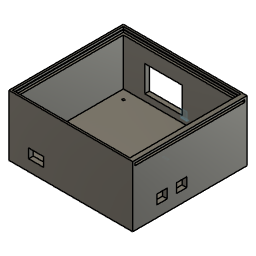
Shades+PCB+Holder+#1 (Autodesk Fusion 360 design; units mm, degrees)
Autodesk Fusion 360 part; units mm, degrees
sketch "Sketch1" plane through (0, 0, 0) normal (0, 1, 0) x (1, 0, 0)
  line L0 (0, 0) -> (132.5, 0)
  line L1 (132.5, 0) -> (132.5, 122.5)
  line L2 (132.5, 122.5) -> (0, 122.5)
  line L3 (0, 122.5) -> (0, 0)
  line L4 (127.5, 117.5) -> (5, 117.5)
  line L5 (5, 117.5) -> (5, 5)
  line L6 (5, 5) -> (127.5, 5)
  line L7 (127.5, 5) -> (127.5, 117.5)
  constraint coincident L0.start L3.end
  constraint horizontal L0
  constraint perpendicular L0 L1
  constraint perpendicular L1 L2
  constraint perpendicular L0 L3
  constraint horizontal L4
  constraint vertical L5
  constraint horizontal L6
  constraint vertical L7
extrude "Extrude1" add sketch "Sketch1" along normal blind 5 contours L0 L1 L2 L3 | L4 L5 L6 L7
sketch "Sketch2" plane through (0, 5, 0) normal (0, 1, 0) x (-1, 0, 0)
  line L0 (0, -122.5) -> (0, 0)
  line L1 (0, 0) -> (-132.5, 0)
  line L2 (-132.5, 0) -> (-132.5, -122.5)
  line L3 (-132.5, -122.5) -> (0, -122.5)
  line L4 (0, -122.5) -> (-5, -122.5)
  line L5 (-132.5, 0) -> (-127.5, 0)
  line L6 (-5, -117.5) -> (-127.5, -117.5)
  line L7 (-127.5, -117.5) -> (-127.5, -5)
  line L8 (-127.5, -5) -> (-5, -5)
  line L9 (-5, -5) -> (-5, -117.5)
  dimension "d19" = 5
  dimension "d20" = 5
  constraint coincident L0.start L3.end
  constraint coincident L3 L4.end
  constraint perpendicular L0 L4
  constraint coincident L1.end L2.start
  constraint perpendicular L2 L5
  constraint horizontal L6
  constraint vertical L7
  constraint horizontal L8
  constraint vertical L9
  measures "d19" distance of L4.end L6.start
  measures "d20" distance of L1.end L5.end
extrude "Extrude2" add sketch "Sketch2" along normal blind 25
sketch "Sketch3" plane through (132.5, 0, 0) normal (1, 0, 0) x (0, 0, -1)
  line L0 (0, 0) -> (122.5, 0)
  line L1 (122.5, 0) -> (122.5, 30)
  line L2 (122.5, 30) -> (0, 30)
  line L3 (0, 30) -> (0, 0)
  circle A0 centre (20, 15) radius 2.5
  circle A1 centre (35, 15) radius 2.5
  line L4 (20, 15) -> (20, 17.5)
  line L5 (20, 17.5) -> (16, 17.5)
  line L6 (20, 15) -> (20, 12.5)
  line L7 (20, 12.5) -> (24, 12.5)
  line L8 (16, 17.5) -> (24, 17.5)
  line L9 (24, 17.5) -> (24, 12.5)
  line L10 (24, 12.5) -> (16, 12.5)
  line L11 (16, 12.5) -> (16, 17.5)
  line L12 (35, 15) -> (35, 17.5)
  line L13 (35, 17.5) -> (31, 17.5)
  line L14 (35, 12.5) -> (39, 12.5)
  line L15 (31, 17.5) -> (39, 17.5)
  line L16 (39, 17.5) -> (39, 12.5)
  line L17 (39, 12.5) -> (31, 12.5)
  line L18 (31, 12.5) -> (31, 17.5)
  line L19 (0, 30) -> (0, 27.5)
  line L20 (0, 27.5) -> (2.5, 27.5)
  line L21 (2.5, 27.5) -> (2.5, 25)
  line L22 (122.5, 30) -> (122.5, 27.5)
  line L23 (122.5, 27.5) -> (120, 27.5)
  line L24 (120, 27.5) -> (120, 25)
  line L25 (120, 25) -> (2.5, 25)
  line L26 (2.5, 27.5) -> (120, 27.5)
  dimension "d23" = 5
  dimension "d24" = 5
  dimension "d58" = 2.5
  dimension "d59" = 2.5
  dimension "d60" = 2.5
  dimension "d61" = 2.5
  constraint coincident A0.centre L4.start
  constraint coincident A0 L4.end
  constraint perpendicular L2 L4
  constraint tangent A0 L5
  constraint coincident A0 L6.end
  constraint perpendicular L5 L6
  constraint tangent A0 L7
  constraint horizontal L8
  constraint vertical L9
  constraint horizontal L10
  constraint vertical L11
  constraint coincident A1.centre L12.start
  constraint coincident A1 L12.end
  constraint perpendicular L2 L12
  constraint tangent A1 L13
  constraint coincident A1 L14.start
  constraint tangent A1 L14
  constraint perpendicular L12 L14
  constraint horizontal L15
  constraint vertical L16
  constraint horizontal L17
  constraint vertical L18
  constraint coincident L2.end L3.start
  constraint perpendicular L2 L19
  constraint perpendicular L19 L20
  constraint perpendicular L20 L21
  constraint coincident L1.end L2.start
  constraint perpendicular L2 L22
  constraint perpendicular L22 L23
  constraint perpendicular L23 L24
  constraint perpendicular L24 L25
  measures "d23" diameter of A0
  measures "d24" diameter of A1
  measures "d58" distance of L2.end L19.end
  measures "d59" distance of L19.end L20.end
  measures "d60" distance of L1.end L22.end
  measures "d61" distance of L22.end L23.end
extrude "Extrude3" cut sketch "Sketch3" against normal blind 10 contours A1
extrude "Extrude4" cut sketch "Sketch3" against normal blind 10 contours A0 L4 L6 | A0 L4 L6
sketch "Sketch4" plane through (0, 0, 0) normal (0, 0, 1) x (1, 0, 0)
  line L0 (0, 0) -> (132.5, 0)
  line L1 (132.5, 0) -> (132.5, 30)
  line L2 (132.5, 30) -> (0, 30)
  line L3 (0, 30) -> (0, 0)
  circle A0 centre (15, 15) radius 3.75
  line L4 (15, 15) -> (15, 18.75)
  line L5 (15, 18.75) -> (10, 18.75)
  line L6 (15, 15) -> (15, 11.25)
  line L7 (15, 11.25) -> (20, 11.25)
  line L8 (10, 18.75) -> (20, 18.75)
  line L9 (20, 18.75) -> (20, 11.25)
  line L10 (20, 11.25) -> (10, 11.25)
  line L11 (10, 11.25) -> (10, 18.75)
  dimension "d29" = 7.5
  constraint coincident A0.centre L4.start
  constraint coincident A0 L4.end
  constraint perpendicular L2 L4
  constraint tangent A0 L5
  constraint coincident A0 L6.end
  constraint perpendicular L5 L6
  constraint tangent A0 L7
  constraint horizontal L8
  constraint vertical L9
  constraint horizontal L10
  constraint vertical L11
  measures "d29" diameter of A0
extrude "Extrude5" cut sketch "Sketch4" against normal blind 10 contours A0 L4 L6 | A0 L4 L6
sketch "Sketch5" plane through (0, 5, 0) normal (0, 1, 0) x (-1, 0, 0)
  line L0 (-127.5, -5) -> (-127.5, -117.5)
  line L1 (-127.5, -117.5) -> (-5, -117.5)
  line L2 (-5, -117.5) -> (-5, -5)
  line L3 (-5, -5) -> (-127.5, -5)
  line L4 (-127.5, -117.5) -> (-86.9, -117.5)
  line L5 (-86.9, -117.5) -> (-86.9, -101.5)
  line L6 (-86.9, -101.5) -> (-86.9, -102.5)
  line L7 (-86.9, -102.5) -> (-84.4, -102.5)
  line L8 (-86.9, -101.5) -> (-86.9, -100.5)
  line L9 (-86.9, -100.5) -> (-89.4, -100.5)
  line L10 (-84.4, -102.5) -> (-89.4, -102.5)
  line L11 (-89.4, -102.5) -> (-89.4, -100.5)
  line L12 (-89.4, -100.5) -> (-84.4, -100.5)
  line L13 (-84.4, -100.5) -> (-84.4, -102.5)
  line L14 (-84.4, -102.5) -> (-83.4, -102.5)
  line L15 (-84.4, -100.5) -> (-83.4, -100.5)
  line L16 (-83.4, -102.5) -> (-83.4, -100.5)
  line L17 (-89.4, -102.5) -> (-90.4, -102.5)
  line L18 (-89.4, -100.5) -> (-90.4, -100.5)
  line L19 (-90.4, -102.5) -> (-90.4, -100.5)
  line L20 (-86.9, -101.5) -> (-86.9, -81)
  line L21 (-86.9, -81) -> (-86.9, -82)
  line L22 (-86.9, -81) -> (-86.9, -80)
  line L23 (-86.9, -82) -> (-83.9, -82)
  line L24 (-83.9, -82) -> (-83.9, -81)
  line L25 (-86.9, -82) -> (-89.9, -82)
  line L26 (-89.9, -82) -> (-89.9, -80)
  line L27 (-89.9, -80) -> (-83.9, -80)
  line L28 (-83.9, -80) -> (-83.9, -81)
  line L29 (-86.9, -81) -> (-86.9, -80)
  dimension "d32" = 40.6
  dimension "d36" = 16
  dimension "d37" = 1
  dimension "d38" = 2.5
  dimension "d39" = 1
  dimension "d40" = 2.5
  dimension "d41" = 1
  dimension "d42" = 1
  dimension "d43" = 1
  dimension "d44" = 1
  dimension "d45" = 20.5
  dimension "d46" = 1
  dimension "d47" = 3
  dimension "d48" = 3
  constraint coincident L0.end L1.start
  constraint perpendicular L0 L4
  constraint perpendicular L4 L5
  constraint vertical L6
  constraint perpendicular L5 L7
  constraint perpendicular L7 L8
  constraint perpendicular L8 L9
  constraint horizontal L10
  constraint vertical L11
  constraint horizontal L12
  constraint vertical L13
  constraint perpendicular L13 L14
  constraint perpendicular L13 L15
  constraint perpendicular L11 L17
  constraint perpendicular L11 L18
  constraint perpendicular L12 L20
  constraint parallel L20 L21
  constraint parallel L21 L22
  constraint perpendicular L20 L23
  constraint perpendicular L23 L24
  constraint perpendicular L20 L25
  constraint perpendicular L25 L26
  constraint perpendicular L26 L27
  constraint parallel L24 L28
  measures "d32" distance of L0.end L4.end
  measures "d36" distance of L4.end L5.end
  measures "d37" distance of L5.end L6.end
  measures "d38" distance of L6.end L7.end
  measures "d39" distance of L5.end L8.end
  measures "d40" distance of L8.end L9.end
  measures "d41" distance of L7.end L14.end
  measures "d42" distance of L12.end L15.end
  measures "d43" distance of L10.end L17.end
  measures "d44" distance of L9.end L18.end
  measures "d45" distance of L5.end L20.end
  measures "d46" distance of L20.end L21.end
  measures "d47" distance of L21.end L23.end
  measures "d48" distance of L21.end L25.end
extrude "Extrude6" add sketch "Sketch5" along normal blind 5 contours L0 L1 L2 L3 L4 | L5 L6 L8 L9 L10 L11 L12 L20 | L5 L6 L7 L8 L10 L12 L13 L20 | L13 L14 L15 L16 | L11 L17 L18 L19 | L20 L21 L22 L25 L26 L27 L29 | L20 L21 L22 L23 L24 L27 L28 L29
extrude "Extrude7" cut 1 faces at (86.6667, 10, -42.5) along direction (0, -1, 0) blind 5
move_face "OffsetFaces1" offset 5 1 faces at (44.1667, 0, -40.8333)
extrude "Extrude8" cut sketch "Sketch5" against normal blind 9 contours L5 L6 L8 L9 L10 L11 L12 L20 | L5 L6 L7 L8 L10 L12 L13 L20 | L13 L14 L15 L16 | L11 L17 L18 L19 | L20 L21 L22 L25 L26 L27 L29 | L20 L21 L22 L23 L24 L27 L28 L29
extrude "Extrude9" cut sketch "Sketch4" against normal blind 10 contours A0 L7 L8 L9 L10 | A0 L5 L8 L10 L11
extrude "Extrude10" cut sketch "Sketch3" against normal blind 15 contours A0 L7 L8 L9 L10 | A0 L5 L8 L10 L11 | A1 L14 L15 L16 L17 | A1 L13 L15 L17 L18
extrude "Extrude11" cut sketch "Sketch3" against normal blind 130 contours L21 L24 L25 L26
sketch "Sketch6" plane through (0, 5, 0) normal (0, 1, 0) x (-1, 0, 0)
  line L0 (-83.4, -100.5) -> (-83.4, -102.5)
  line L1 (-83.4, -102.5) -> (-90.4, -102.5)
  line L2 (-90.4, -102.5) -> (-90.4, -100.5)
  line L3 (-90.4, -100.5) -> (-83.4, -100.5)
  line L4 (-83.9, -80) -> (-83.9, -82)
  line L5 (-83.9, -82) -> (-89.9, -82)
  line L6 (-89.9, -82) -> (-89.9, -80)
  line L7 (-89.9, -80) -> (-83.9, -80)
  line L8 (-127.5, -117.5) -> (-5, -117.5)
  line L9 (-5, -117.5) -> (-5, -5)
  line L10 (-5, -5) -> (-127.5, -5)
  line L11 (-127.5, -5) -> (-127.5, -117.5)
  line L12 (-127.5, -117.5) -> (-117.5, -117.5)
  line L13 (-117.5, -117.5) -> (-117.5, -107.5)
  circle A0 centre (-117.5, -107.5) radius 1.25
  line L14 (-117.5, -107.5) -> (-117.5, -14.9)
  line L15 (-117.5, -14.9) -> (-15.1, -14.9)
  line L16 (-15.1, -14.9) -> (-15.1, -107.5)
  line L17 (-15.1, -107.5) -> (-117.5, -107.5)
  circle A1 centre (-117.5, -14.9) radius 1.25
  circle A2 centre (-15.1, -14.9) radius 1.25
  circle A3 centre (-15.1, -107.5) radius 1.25
  dimension "d64" = 10
  dimension "d65" = 10
  dimension "d66" = 2.5
  dimension "d67" = 92.6
  dimension "d68" = 102.4
  dimension "d69" = 92.6
  dimension "d70" = 2.5
  dimension "d71" = 2.5
  dimension "d72" = 2.5
  constraint coincident L8.start L11.end
  constraint perpendicular L11 L12
  constraint perpendicular L8 L13
  constraint coincident L13.end A0.centre
  constraint perpendicular L10 L14
  constraint perpendicular L14 L15
  constraint perpendicular L15 L16
  constraint coincident L14.end L15.start
  constraint coincident L15.end L16.start
  constraint coincident L16.end L17.start
  measures "d64" distance of L8.start L12.end
  measures "d65" distance of L12.end L13.end
  measures "d66" diameter of A0
  measures "d67" distance of L13.end L14.end
  measures "d68" distance of L14.end L15.end
  measures "d69" distance of L15.end L16.end
  measures "d70" diameter of A1
  measures "d71" diameter of A2
  measures "d72" diameter of A3
extrude "Extrude12" add sketch "Sketch6" along normal blind 90 contours L13 A0 L14 | L13 A0 L17 | A0 L14 L17 | L14 L15 A1 | L14 L15 A1 | L16 L17 A3 | L16 L17 A3 | L15 L16 A2 | L15 L16 A2
extrude "Extrude13" cut 4 faces at (15.1927, 95, -108.3757) (117.8443, 95, -107.8589) (117.1946, 95, -14.6166) (14.7696, 95, -14.8502) along direction (0, -1, 0) blind 120
sketch "Sketch7" plane through (0, -5, 0) normal (0, -1, 0) x (1, 0, 0)
  circle A0 centre (117.5, -14.9) radius 1.25
  circle A1 centre (15.1, -107.5) radius 1.25
  circle A2 centre (117.5, -107.5) radius 1.25
  circle A3 centre (15.1, -14.9) radius 1.25
  line L0 (0, 0) -> (0, -122.5)
  line L1 (0, -122.5) -> (132.5, -122.5)
  line L2 (132.5, -122.5) -> (132.5, 0)
  line L3 (132.5, 0) -> (0, 0)
extrude "Extrude14" add sketch "Sketch7" along normal blind 5
extrude "Extrude15" add 1 faces at (49.5062, -10, -46.0816) along direction (0, -1, 0) blind 5
extrude "Extrude16" cut 1 faces at (45.8333, 29.1667, -5) along direction (0, 0, 1) blind 3
extrude "Extrude17" cut 2 faces at (5, 29.1667, -80) (5, 29.1667, -3.1667) along direction (-1, 0, 0) blind 3
extrude "Extrude18" cut 2 faces at (45.8333, 28.3333, -117.5) (3.1667, 29.1667, -117.5) along direction (0, 0, -1) blind 3
sketch "Sketch8" plane through (0, 5, 0) normal (0, 1, 0) x (-1, 0, 0)
  circle A0 centre (-117.5, -14.9) radius 1.25
  circle A1 centre (-15.1, -107.5) radius 1.25
  circle A2 centre (-15.1, -14.9) radius 1.25
  circle A3 centre (-117.5, -107.5) radius 1.25
  line L0 (-83.4, -100.5) -> (-83.4, -102.5)
  line L1 (-83.4, -102.5) -> (-90.4, -102.5)
  line L2 (-90.4, -102.5) -> (-90.4, -100.5)
  line L3 (-90.4, -100.5) -> (-83.4, -100.5)
  line L4 (-83.9, -80) -> (-83.9, -82)
  line L5 (-83.9, -82) -> (-89.9, -82)
  line L6 (-89.9, -82) -> (-89.9, -80)
  line L7 (-89.9, -80) -> (-83.9, -80)
  line L8 (-127.5, -117.5) -> (-5, -117.5)
  line L9 (-5, -117.5) -> (-5, -5)
  line L10 (-5, -5) -> (-127.5, -5)
  line L11 (-127.5, -5) -> (-127.5, -117.5)
sketch "Sketch9" plane through (0, -15, 0) normal (0, -1, 0) x (1, 0, 0)
  circle A0 centre (15.1, -14.9) radius 1.25
  circle A1 centre (117.5, -107.5) radius 1.25
  circle A2 centre (117.5, -14.9) radius 1.25
  circle A3 centre (15.1, -107.5) radius 1.25
  line L0 (132.5, 0) -> (0, 0)
  line L1 (0, 0) -> (0, -122.5)
  line L2 (0, -122.5) -> (132.5, -122.5)
  line L3 (132.5, -122.5) -> (132.5, 0)
extrude "Extrude19" add sketch "Sketch9" along normal blind 25
extrude "Extrude20" cut 1 faces at (49.5062, -40, -46.0816) along direction (0, 1, 0) blind 5
sketch "Sketch10" plane through (0, 5, 0) normal (0, 1, 0) x (-1, 0, 0)
extrude "Extrude21" cut sketch "Sketch8" against normal blind 35 contours L4 L5 L6 L7
sketch "Sketch11" plane through (0, -30, 0) normal (0, 1, 0) x (-1, 0, 0)
  line L0 (-89.9, -80) -> (-89.9, -82)
  line L1 (-89.9, -82) -> (-83.9, -82)
  line L2 (-83.9, -82) -> (-83.9, -80)
  line L3 (-83.9, -80) -> (-89.9, -80)
sketch "Sketch12" plane through (0, -30, 0) normal (0, 1, 0) x (-1, 0, 0)
sketch "Sketch13" plane through (0, -4, 0) normal (0, 1, 0) x (-1, 0, 0)
  line L0 (-90.4, -102.5) -> (-83.4, -102.5)
  line L1 (-83.4, -102.5) -> (-83.4, -100.5)
  line L2 (-83.4, -100.5) -> (-90.4, -100.5)
  line L3 (-90.4, -100.5) -> (-90.4, -102.5)
sketch "Sketch14" plane through (0, 0, -100.5) normal (0, 0, -1) x (-1, 0, 0)
  line L0 (-83.4, 5) -> (-90.4, 5)
  line L1 (-90.4, 5) -> (-90.4, -4)
  line L2 (-90.4, -4) -> (-83.4, -4)
  line L3 (-83.4, -4) -> (-83.4, 5)
sketch "Sketch15" plane through (0, 5, 0) normal (0, 1, 0) x (-1, 0, 0)
  circle A0 centre (-117.5, -14.9) radius 1.25
  circle A1 centre (-15.1, -107.5) radius 1.25
  circle A2 centre (-15.1, -14.9) radius 1.25
  circle A3 centre (-117.5, -107.5) radius 1.25
  line L0 (-83.4, -100.5) -> (-83.4, -102.5)
  line L1 (-83.4, -102.5) -> (-90.4, -102.5)
  line L2 (-90.4, -102.5) -> (-90.4, -100.5)
  line L3 (-90.4, -100.5) -> (-83.4, -100.5)
  line L4 (-83.9, -80) -> (-83.9, -82)
  line L5 (-83.9, -82) -> (-89.9, -82)
  line L6 (-89.9, -82) -> (-89.9, -80)
  line L7 (-89.9, -80) -> (-83.9, -80)
  line L8 (-127.5, -117.5) -> (-5, -117.5)
  line L9 (-5, -117.5) -> (-5, -5)
  line L10 (-5, -5) -> (-127.5, -5)
  line L11 (-127.5, -5) -> (-127.5, -117.5)
sketch "Sketch16" plane through (0, 5, 0) normal (0, 1, 0) x (-1, 0, 0)
extrude "Extrude22" cut sketch "Sketch15" against normal blind 35 contours L0 L1 L2 L3
sketch "Sketch17" plane through (0, 5, 0) normal (0, 1, 0) x (-1, 0, 0)
  circle A0 centre (-117.5, -14.9) radius 1.25
  circle A1 centre (-15.1, -107.5) radius 1.25
  circle A2 centre (-15.1, -14.9) radius 1.25
  circle A3 centre (-117.5, -107.5) radius 1.25
  line L0 (-83.4, -100.5) -> (-83.4, -102.5)
  line L1 (-83.4, -102.5) -> (-90.4, -102.5)
  line L2 (-90.4, -102.5) -> (-90.4, -100.5)
  line L3 (-90.4, -100.5) -> (-83.4, -100.5)
  line L4 (-83.9, -80) -> (-83.9, -82)
  line L5 (-83.9, -82) -> (-89.9, -82)
  line L6 (-89.9, -82) -> (-89.9, -80)
  line L7 (-89.9, -80) -> (-83.9, -80)
  line L8 (-127.5, -117.5) -> (-5, -117.5)
  line L9 (-5, -117.5) -> (-5, -5)
  line L10 (-5, -5) -> (-127.5, -5)
  line L11 (-127.5, -5) -> (-127.5, -117.5)
extrude "Extrude23" cut sketch "Sketch17" against normal blind 30
sketch "Sketch18" plane through (0, 0, 0) normal (0, 0, 1) x (1, 0, 0)
  line L0 (0, -35) -> (132.5, -35)
  line L1 (132.5, -35) -> (132.5, 30)
  line L2 (132.5, 30) -> (0, 30)
  line L3 (0, 30) -> (0, -35)
  line L4 (10, 18.75) -> (20, 18.75)
  line L5 (20, 18.75) -> (20, 11.25)
  line L6 (20, 11.25) -> (10, 11.25)
  line L7 (10, 11.25) -> (10, 18.75)
sketch "Sketch19" plane through (132.5, 0, 0) normal (1, 0, 0) x (0, 0, -1)
  line L0 (0, -35) -> (122.5, -35)
  line L1 (122.5, -35) -> (122.5, 30)
  line L2 (122.5, 30) -> (0, 30)
  line L3 (0, 30) -> (0, -35)
  line L4 (120, 25) -> (2.5, 25)
  line L5 (2.5, 25) -> (2.5, 27.5)
  line L6 (2.5, 27.5) -> (120, 27.5)
  line L7 (120, 27.5) -> (120, 25)
  line L8 (16, 17.5) -> (24, 17.5)
  line L9 (24, 17.5) -> (24, 12.5)
  line L10 (24, 12.5) -> (16, 12.5)
  line L11 (16, 12.5) -> (16, 17.5)
  line L12 (31, 17.5) -> (39, 17.5)
  line L13 (39, 17.5) -> (39, 12.5)
  line L14 (39, 12.5) -> (31, 12.5)
  line L15 (31, 12.5) -> (31, 17.5)
  line L16 (26, -23) -> (37, -23)
  line L17 (37, -23) -> (37, -13)
  line L18 (37, -13) -> (26, -13)
  line L19 (26, -13) -> (26, -23)
  line L20 (47, -23) -> (58, -23)
  line L21 (58, -23) -> (58, -13)
  line L22 (58, -13) -> (47, -13)
  line L23 (47, -13) -> (47, -23)
  constraint horizontal L16
  constraint vertical L17
  constraint horizontal L18
  constraint vertical L19
  constraint horizontal L20
  constraint vertical L21
  constraint horizontal L22
  constraint vertical L23
extrude "Extrude24" cut sketch "Sketch19" against normal blind 5 contours L16 L17 L18 L19
sketch "Sketch20" plane through (132.5, 0, 0) normal (1, 0, 0) x (0, 0, -1)
  line L0 (37, -23) -> (26, -23)
  line L1 (26, -23) -> (26, -13)
  line L2 (26, -13) -> (37, -13)
  line L3 (37, -13) -> (37, -23)
  line L4 (0, -35) -> (122.5, -35)
  line L5 (122.5, -35) -> (122.5, 30)
  line L6 (122.5, 30) -> (0, 30)
  line L7 (0, 30) -> (0, -35)
  line L8 (120, 25) -> (2.5, 25)
  line L9 (2.5, 25) -> (2.5, 27.5)
  line L10 (2.5, 27.5) -> (120, 27.5)
  line L11 (120, 27.5) -> (120, 25)
  line L12 (16, 17.5) -> (24, 17.5)
  line L13 (24, 17.5) -> (24, 12.5)
  line L14 (24, 12.5) -> (16, 12.5)
  line L15 (16, 12.5) -> (16, 17.5)
  line L16 (31, 17.5) -> (39, 17.5)
  line L17 (39, 17.5) -> (39, 12.5)
  line L18 (39, 12.5) -> (31, 12.5)
  line L19 (31, 12.5) -> (31, 17.5)
  line L20 (47, -23) -> (58, -23)
  line L21 (58, -23) -> (58, -13)
  line L22 (58, -13) -> (47, -13)
  line L23 (47, -13) -> (47, -23)
  constraint horizontal L20
  constraint vertical L21
  constraint horizontal L22
  constraint vertical L23
extrude "Extrude25" cut sketch "Sketch20" against normal blind 5 contours L20 L21 L22 L23
sketch "Sketch21" plane through (0, 0, 0) normal (0, 0, 1) x (1, 0, 0)
sketch "Sketch22" plane through (0, 0, 0) normal (0, 0, 1) x (1, 0, 0)
sketch "Sketch23" plane through (132.5, 0, 0) normal (1, 0, 0) x (0, 0, -1)
  line L0 (58, -23) -> (47, -23)
  line L1 (47, -23) -> (47, -13)
  line L2 (47, -13) -> (58, -13)
  line L3 (58, -13) -> (58, -23)
  line L4 (37, -23) -> (26, -23)
  line L5 (26, -23) -> (26, -13)
  line L6 (26, -13) -> (37, -13)
  line L7 (37, -13) -> (37, -23)
  line L8 (0, -35) -> (122.5, -35)
  line L9 (122.5, -35) -> (122.5, 30)
  line L10 (122.5, 30) -> (0, 30)
  line L11 (0, 30) -> (0, -35)
  line L12 (120, 25) -> (2.5, 25)
  line L13 (2.5, 25) -> (2.5, 27.5)
  line L14 (2.5, 27.5) -> (120, 27.5)
  line L15 (120, 27.5) -> (120, 25)
  line L16 (16, 17.5) -> (24, 17.5)
  line L17 (24, 17.5) -> (24, 12.5)
  line L18 (24, 12.5) -> (16, 12.5)
  line L19 (16, 12.5) -> (16, 17.5)
  line L20 (31, 17.5) -> (39, 17.5)
  line L21 (39, 17.5) -> (39, 12.5)
  line L22 (39, 12.5) -> (31, 12.5)
  line L23 (31, 12.5) -> (31, 17.5)
sketch "Sketch24" plane through (0, 0, 0) normal (0, 0, 1) x (1, 0, 0)
  line L0 (21, -23) -> (37, -23)
  line L1 (37, -23) -> (37, -13)
  line L2 (37, -13) -> (21, -13)
  line L3 (21, -13) -> (21, -23)
  constraint horizontal L0
  constraint vertical L1
  constraint horizontal L2
  constraint vertical L3
extrude "Extrude26" cut sketch "Sketch24" against normal blind 5
extrude "Extrude27" add sketch "Sketch18" against normal blind 5 contours L4 L5 L6 L7
extrude "Extrude28" add sketch "Sketch23" against normal blind 5 contours L16 L17 L18 L19
sketch "Sketch25" plane through (132.5, 0, 0) normal (1, 0, 0) x (0, 0, -1)
  line L0 (58, -23) -> (47, -23)
  line L1 (47, -23) -> (47, -13)
  line L2 (47, -13) -> (58, -13)
  line L3 (58, -13) -> (58, -23)
  line L4 (37, -23) -> (26, -23)
  line L5 (26, -23) -> (26, -13)
  line L6 (26, -13) -> (37, -13)
  line L7 (37, -13) -> (37, -23)
  line L8 (0, -35) -> (122.5, -35)
  line L9 (122.5, -35) -> (122.5, 30)
  line L10 (122.5, 30) -> (0, 30)
  line L11 (0, 30) -> (0, -35)
  line L12 (120, 25) -> (2.5, 25)
  line L13 (2.5, 25) -> (2.5, 27.5)
  line L14 (2.5, 27.5) -> (120, 27.5)
  line L15 (120, 27.5) -> (120, 25)
  line L16 (31, 17.5) -> (39, 17.5)
  line L17 (39, 17.5) -> (39, 12.5)
  line L18 (39, 12.5) -> (31, 12.5)
  line L19 (31, 12.5) -> (31, 17.5)
extrude "Extrude29" add sketch "Sketch25" against normal blind 5 contours L16 L17 L18 L19
sketch "Sketch26" plane through (0, 0, -122.5) normal (0, 0, -1) x (-1, 0, 0)
  line L0 (-132.5, -35) -> (0, -35)
  line L1 (0, -35) -> (0, 30)
  line L2 (0, 30) -> (-132.5, 30)
  line L3 (-132.5, 30) -> (-132.5, -35)
  line L4 (-28, -22) -> (-68, -22)
  line L5 (-68, -22) -> (-68, 10)
  line L6 (-68, 10) -> (-28, 10)
  line L7 (-28, 10) -> (-28, -22)
  constraint horizontal L4
  constraint vertical L5
  constraint horizontal L6
  constraint vertical L7
sketch "Sketch27" plane through (0, 0, -122.5) normal (0, 0, -1) x (-1, 0, 0)
extrude "Extrude30" cut sketch "Sketch26" against normal blind 5 contours L4 L5 L6 L7
extrude "Extrude31" add 1 faces at (41.3333, -22, -120.8333) along direction (0, 1, 0) blind 4
